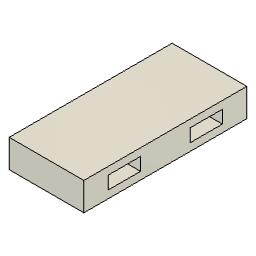
Parametric Centerpiece Template Pin Holes (Autodesk Fusion 360 design; units mm, degrees)
Autodesk Fusion 360 part; units mm, degrees
sketch "Sketch1" plane through (0, 0, 0) normal (0, -1, 0) x (1, 0, 0) in component "DDD Wall Control Center Piece Parametric Template"
  line L0 (11.6, -25.3) -> (-11.6, -25.3)
  line L1 (-11.6, -25.3) -> (-11.6, 25.3)
  line L2 (-11.6, 25.3) -> (11.6, 25.3)
  line L3 (11.6, 25.3) -> (11.6, -25.3)
  line L4 (11.6, -25.3) -> (-11.6, 25.3) construction
  line L5 (-11.6, -25.3) -> (11.6, 25.3) construction
  dimension "d1" = 23.2
  dimension "d2" = 50.6
  constraint horizontal L0
  constraint perpendicular L0 L1
  constraint parallel L0 L2
  constraint parallel L1 L3
  constraint coincident L4 origin
  constraint coincident L5 origin
  constraint vertical L1
  measures "d1" distance of L1.end L2.end
  measures "d2" distance of L0.end L1.end
extrude "Extrude1" add sketch "Sketch1" against normal blind 8.7 in component "DDD Wall Control Center Piece Parametric Template"
sketch "Sketch3" plane through (0, 0, 0) normal (1, 0, 0) x (0, 0, 1) in component "DDD Wall Control Center Piece Parametric Template"
  line L0 (-17.7, -2.35) -> (-7.7, -2.35)
  line L1 (-7.7, -2.35) -> (-7.7, -6.35)
  line L2 (-7.7, -6.35) -> (-17.7, -6.35)
  line L3 (-17.7, -6.35) -> (-17.7, -2.35)
  line L4 (-17.7, -2.35) -> (-7.7, -6.35) construction
  line L5 (-7.7, -2.35) -> (-17.7, -6.35) construction
  line L6 (1.75, 0) -> (22.5, 0)
  line L7 (25.3, 0) -> (-25.3, 0)
  point P0 (-12.7, -4.35)
  dimension "d165" = 10
  dimension "d166" = 4
  dimension "d189" = 17.7
  dimension "d205" = 2.35
  constraint horizontal L0
  constraint perpendicular L0 L1
  constraint parallel L0 L2
  constraint parallel L1 L3
  constraint coincident L4 P0
  constraint coincident L5 P0
  measures "d165" distance of L1.end L2.end
  measures "d166" distance of L0.start L2.end
  measures "d189" distance of origin L3
  measures "d205" distance of L0 L7
extrude "Extrude3" cut sketch "Sketch3" against normal blind 4 from surface at 11.6 in component "DDD Wall Control Center Piece Parametric Template"
mirror "Mirror2" about plane through (0, 0, 0) normal (1, 0, 0) of "Extrude3" in component "DDD Wall Control Center Piece Parametric Template"
pattern_linear "R-Pattern4" count 2 spacing 25.4 along (0, 0, 1) of "Extrude3" in component "DDD Wall Control Center Piece Parametric Template"
mirror "Mirror1" about plane through (0, 0, 0) normal (1, 0, 0) of "R-Pattern4" in component "DDD Wall Control Center Piece Parametric Template"
component "DDD Wall Control Center Piece Parametric Template" placed x (1, 0, 0) y (0, 1, 0) z (0, 0, 1) at (0, 0, 0)
equation "d1 = HorizontalWidth"
equation "d2 = VerticalHeight"
equation "d3 = -Depth"
equation "d42 = -PinHoleWidth / 2"
equation "HowToUse = 0" comment "Save this as a new design   from the original to preserve the template.  Then modify as needed for centerpiece divider racks."
equation "d165 = PinHoleLength"
equation "d166 = PinHoleHeight"
equation "d168 = VerticalUnits"
equation "d170 = -SlotSpacing"
equation "HorizontalUnits = 1" comment "Units spanning horizontally across the wall control board/pegboard"
equation "VerticalUnits = 2" comment "Units spanning vertically down the wall control board/pegboard"
equation "SidepieceDepth = 8.7 mm" comment "Sidepiece depth used to ensure the spaces for the pins line up"
equation "HorizontalWidthBetweenSlots = SlotSpacing - SlotWidth" comment "The space between two slots in a wall control board"
equation "PinHoleLength = 10 mm"
equation "PinHoleWidth = 8 mm"
equation "PinHoleHeight = 4 mm"
equation "SlotSpacing = 25.4 mm" comment "Slots in wall control boards are spaced an inch apart"
equation "PinToEdgeLength = 7.6 mm" comment "Distance from the back edge of the center piece to the first pin"
equation "HorizontalWidth = ( HorizontalUnits - 1 ) * SlotSpacing + HorizontalWidthBetweenSlots"
equation "VerticalHeight = ( VerticalUnits - 1 ) * SlotSpacing + PinHoleLength + 2 * PinToEdgeLength"
equation "d189 = ( VerticalHeight / 2 ) - PinToEdgeLength"
equation "Depth = max(DepthOverride; PinHoleHeight + PinDepthOffset * 2)"
equation "SlotWidth = 2.2 mm"
equation "DepthOverride = 0 mm" comment "Add additional depth to the centerpiece. There is an enforced minimum to allow for the pins."
equation "PinDepthOffset = ( SidepieceDepth - PinHoleHeight ) / 2"
equation "d205 = PinDepthOffset"
named bodies: "Center Piece Parametric Template"
